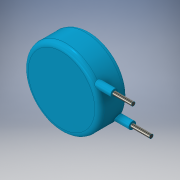
# Autodesk Inventor part: 16mm_7_2mmDiskPTC
Saved by Autodesk Inventor 2016 (Build 200138000, 138)
## iProperties
Created: 2016-09-30
Part Number: 16mm_7_2mmDiskPTC
Material: Generic
Document SubType Name: Modeling
Designer: jfixelle
Density: 1 g/cm^3
Appearance: Sky Blue Dark
Author: jfixelle
Autodesk Inventor part; units mm, degrees
ref_plane "YZ Plane" through (0, 0, 0) normal (1, 0, 0) x (0, 1, 0)
ref_plane "XZ Plane" through (0, 0, 0) normal (0, 1, 0) x (-1, 0, 0)
ref_plane "XY Plane" through (0, 0, 0) normal (0, 0, 1) x (1, 0, 0)
sketch "Sketch1" plane through (0, 0, 0) normal (0, 0, 1) x (1, 0, 0)
  circle A0 centre (0, 0) radius 8
  dimension "d0" = 16
  constraints: 1 centre point, 1 coincident
  measures "d0" diameter of A0
extrude "Extrusion1" add sketch "Sketch1" along normal mid plane 6
fillet "Fillet1" radius 1 2 edges at (-8, 0, 3) (-8, 0, -3)
sketch "Sketch2" plane through (0, 0, 0) normal (1, 0, 0) x (0, 1, 0)
  circle A0 centre (3.9, 1.9) radius 0.75
  circle A1 centre (-3.9, -1.9) radius 0.75
  point P0 (0, 0)
  dimension "d4" = 3.9
  dimension "d5" = 3.9
  dimension "d8" = 1.5
  dimension "d9" = 1.5
  dimension "d20" = 1.9
  dimension "d21" = 1.9
  constraints: 2 centre point
  measures "d4" horizontal distance of point (0, 0) A1.centre
  measures "d5" horizontal distance of point (0, 0) A0.centre
  measures "d8" diameter of A0
  measures "d9" diameter of A1
  measures "d20" vertical distance of point (0, 0) A0.centre
  measures "d21" vertical distance of point (0, 0) A1.centre
extrude "Extrusion2" add sketch "Sketch2" along normal blind 10
sketch "Sketch3" plane through (10, 3.9, 1.9) normal (1, 0, 0) x (0, 0, -1)
  circle A0 centre (0, 0) radius 0.4
  circle A1 centre (3.8, -7.8) radius 0.4
  point P0 (1.9, -3.9)
  dimension "d14" = 3.9
  dimension "d15" = 3.9
  dimension "d16" = 0.8
  dimension "d17" = 0.8
  dimension "d22" = 1.9
  dimension "d23" = 1.9
  constraints: 2 centre point
  measures "d14" vertical distance of point (1.9, -3.9) A1.centre
  measures "d15" vertical distance of point (1.9, -3.9) A0.centre
  measures "d16" diameter of A1
  measures "d17" diameter of A0
  measures "d22" horizontal distance of point (1.9, -3.9) A0.centre
  measures "d23" horizontal distance of point (1.9, -3.9) A1.centre
extrude "Extrusion3" add sketch "Sketch3" along normal blind 4
body "Solid1"
